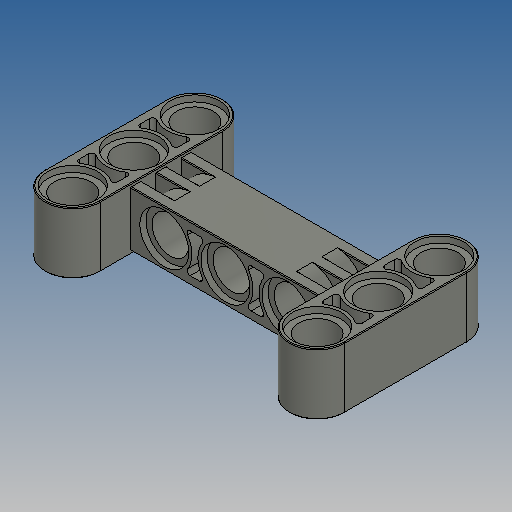
# Autodesk Inventor part: 14720-DkBluishGray
Saved by Autodesk Inventor 2025 (Build 290162010, 162A)
## iProperties
Created: 2012-03-21
Part Number: 14720-DkBluishGray
Document SubType Name: Modeling
Designer: D. Kohfeld
Density: 1.06 g/cm^3
Material: ABS Plastic
Mass: 2.24309 g
Surface Area: 36.022 cm^2
Volume: 2.11613 cm^3
Appearance: DkBluishGray
Author: D. Kohfeld
Autodesk Inventor part; units mm, degrees
ref_plane "YZ Plane" through (0, 0, 0) normal (1, 0, 0) x (0, 1, 0)
ref_plane "XZ Plane" through (0, 0, 0) normal (0, 1, 0) x (-1, 0, 0)
ref_plane "XY Plane" through (0, 0, 0) normal (0, 0, 1) x (1, 0, 0)
sketch "Sketch1" plane through (0, 0, 0) normal (0, 0, 1) x (1, 0, 0)
  line L0 (19.6, -8) -> (19.6, 8)
  line L1 (12.4, 8) -> (12.4, -8)
  arc A0 (19.6, 8) -> (12.4, 8) centre (16, 8) ccw
  arc A1 (12.4, -8) -> (19.6, -8) centre (16, -8) ccw
  circle A2 centre (16, 8) radius 3.2
  circle A3 centre (16, 8) radius 2.4
  line L2 (18.5456, 5.4544) -> (18.5456, 2.5456)
  line L3 (13.4544, 5.4544) -> (13.4544, 2.5456)
  arc A4 (13.4544, 5.4544) -> (18.5456, 5.4544) centre (16, 8) ccw
  arc A5 (18.5456, 2.5456) -> (13.4544, 2.5456) centre (16, 0) ccw
  circle A6 centre (16, 0) radius 3.2
  circle A7 centre (16, 0) radius 2.4
  line L4 (16, 8) -> (13.4544, 5.4544) construction
  circle A8 centre (16, -8) radius 3.2
  circle A9 centre (16, -8) radius 2.4
  line L5 (18.5456, -2.5456) -> (18.5456, -5.4544)
  line L6 (13.4544, -5.4544) -> (13.4544, -2.5456)
  arc A10 (13.4544, -2.5456) -> (18.5456, -2.5456) centre (16, 0) ccw
  arc A11 (18.5456, -5.4544) -> (13.4544, -5.4544) centre (16, -8) ccw
  point P0 (0, 0)
  point P1 (12.4, 0)
  dimension "d49" = 6.4
  dimension "d50" = 4.8
  dimension "d51" = 8
  dimension "d116" = 45
  dimension "d119" = 7.2
  dimension "d131" = 16
  constraints: 14 end point, 12 centre point, 12 point on circle, 9 coincident, 8 equal radius, 4 horizontal alignment, 4 tangent, 3 parallel, 3 vertical alignment, 2 vertical, 1 midpoint
  measures "d49" diameter of A2
  measures "d50" diameter of A3
  measures "d51" distance of A0.centre A5.centre
  measures "d116" angle of L4 L1
  measures "d119" diameter of A0
  measures "d131" distance of A6.centre point (0, 0)
extrude "Extrusion1" add sketch "Sketch1" along normal mid plane 8 contours A1 L1 A0 L0 | A2 | L2 A5 L3 A4 | A6 | A8 | L5 A11 L6 A10
sketch "Sketch6" plane through (0, 0, 4) normal (0, 0, 1) x (1, 0, 0)
  circle A0 centre (16, 8) radius 2.4 projected
  circle A1 centre (16, 8) radius 3.2 projected
  line L0 (18.5456, 5.4544) -> (18.5456, 2.5456) projected
  arc A2 (13.4544, 5.4544) -> (18.5456, 5.4544) centre (16, 8) ccw projected
  arc A3 (18.5456, 2.5456) -> (13.4544, 2.5456) centre (16, 0) ccw projected
  line L1 (13.4544, 5.4544) -> (13.4544, 2.5456) projected
  circle A4 centre (16, 0) radius 3.2 projected
  circle A5 centre (16, -8) radius 3.2 projected
  arc A6 (18.5456, -5.4544) -> (13.4544, -5.4544) centre (16, -8) ccw projected
  line L2 (13.4544, -5.4544) -> (13.4544, -2.5456) projected
  arc A7 (13.4544, -2.5456) -> (18.5456, -2.5456) centre (16, 0) ccw projected
  line L3 (18.5456, -2.5456) -> (18.5456, -5.4544) projected
extrude "Extrusion7" cut sketch "Sketch6" against normal blind 0.8 contours A0 | A1 | A4 | A5
extrude "Extrusion8" cut sketch "Sketch6" against normal blind 3.1 contours L0 A3 L1 A2 | A6 L2 A7 L3
mirror "Mirror5" about plane through (0, 0, 0) normal (0, 0, 1) of "Extrusion7", "Extrusion8"
fillet "Fillet2" radius 0.4 16 edges at (13.4544, 5.4544, 2.45) (13.4544, 2.5456, 2.45) (18.5456, 2.5456, 2.45) (18.5456, 5.4544, 2.45) (13.4544, -2.5456, 2.45) (18.5456, -5.4544, 2.45) (18.5456, -2.5456, 2.45) (13.4544, -5.4544, 2.45) (18.5456, -5.4544, -2.45) (18.5456, -2.5456, -2.45) (13.4544, -5.4544, -2.45) (13.4544, -2.5456, -2.45) (13.4544, 2.5456, -2.45) (13.4544, 5.4544, -2.45) (18.5456, 5.4544, -2.45) (18.5456, 2.5456, -2.45)
fillet "Fillet2" radius 0.1 8 edges at (12.4, 0, 4) (16, 11.6, 4) (19.6, 0, 4) (16, -11.6, 4) (16, 11.6, -4) (12.4, 0, -4) (16, -11.6, -4) (19.6, 0, -4)
sketch "Sketch11" plane through (0, 0, 0) normal (0, 1, 0) x (-1, 0, 0)
  line L0 (8, 3.6) -> (-8, 3.6)
  line L1 (-12.4, 1.111) -> (-12.4, -1.111)
  line L2 (-8, -3.6) -> (8, -3.6)
  line L3 (-12.4, -3.9) -> (-12.4, 3.9) projected
  line L4 (0, 3.6) -> (0, -3.6) construction
  arc A0 (-8, 3.6) -> (-8, -3.6) centre (-8, 0) ccw
  line L5 (-11.4243, 1.111) -> (-12.4, 1.111)
  line L6 (-11.4243, -1.111) -> (-12.4, -1.111)
  arc A1 (8, -3.6) -> (8, 3.6) centre (8, 0) ccw
  line L7 (11.4243, 1.111) -> (12.4, 1.111)
  line L8 (12.4, 1.111) -> (12.4, -1.111)
  line L9 (12.4, -1.111) -> (11.4243, -1.111)
  point P0 (-12.4, 0)
  point P1 (0, 0)
  point P2 (12.4, 0)
  point P3 (0, 0)
  dimension "d121" = 7.2
  dimension "d123" = 2.222
  dimension "d132" = 16
  constraints: 18 end point, 8 point on circle, 6 midpoint, 5 parallel, 4 perpendicular, 4 tangent, 3 horizontal alignment, 2 centre point, 2 point on line, 1 coincident
  measures "d121" distance between parallel lines of L2 L0
  measures "d123" distance between parallel lines of L6 L5
  measures "d132" distance of A1.centre A0.centre
extrude "Extrusion13" add sketch "Sketch11" along normal mid plane 8
sketch "Sketch12" plane through (0, -4, 0) normal (0, -1, 0) x (1, 0, 0)
  arc A0 (-8, 3.6) -> (-8, -3.6) centre (-8, 0) ccw projected
  arc A1 (8, -3.6) -> (11.4243, -1.111) centre (8, 0) ccw projected
  line L0 (11.4243, -1.111) -> (12.4, -1.111) projected
  circle A2 centre (8, 0) radius 2.4
  circle A3 centre (8, 0) radius 3.2
  circle A4 centre (0, 0) radius 2.4
  circle A5 centre (0, 0) radius 3.2
  circle A6 centre (-8, 0) radius 2.4
  circle A7 centre (-8, 0) radius 3.2
  line L1 (-8, 0) -> (0, 0) construction
  line L2 (0, 0) -> (8, 0) construction
  arc A8 (8, -3.6) -> (8, 3.6) centre (8, 0) ccw projected
  arc A9 (-8, 3.6) -> (-8, -3.6) centre (-8, 0) ccw projected
  line L3 (-8, -3.6) -> (8, -3.6) projected
  line L4 (-5.4544, 2.5456) -> (-2.5456, 2.5456)
  line L5 (-5.4544, -2.5456) -> (-2.5456, -2.5456)
  line L6 (2.5456, 2.5456) -> (5.4544, 2.5456)
  line L7 (2.5456, -2.5456) -> (5.4544, -2.5456)
  arc A10 (-5.4544, -2.5456) -> (-5.4544, 2.5456) centre (-8, 0) ccw
  arc A11 (-2.5456, 2.5456) -> (-2.5456, -2.5456) centre (0, 0) ccw
  arc A12 (2.5456, -2.5456) -> (2.5456, 2.5456) centre (0, 0) ccw
  arc A13 (5.4544, 2.5456) -> (5.4544, -2.5456) centre (8, 0) ccw
  line L8 (-8, 0) -> (-5.4544, 2.5456) construction
  point P0 (-11.4243, -1.111)
  point P1 (11.4243, 1.111)
  point P2 (-11.4243, 1.111)
  point P3 (-6.8156, -3.3996)
  dimension "d124" = 4.8
  dimension "d125" = 6.4
  dimension "d126" = 45
  constraints: 14 end point, 10 centre point, 9 coincident, 8 equal radius, 8 point on circle, 5 parallel, 3 equal length, 1 collinear, 1 horizontal alignment, 1 other
  measures "d124" diameter of A2
  measures "d125" diameter of A3
  measures "d126" angle of L1 L8
extrude "Extrusion14" cut sketch "Sketch12" against normal through all contours A2 | A4 | A6
extrude "Extrusion15" cut sketch "Sketch12" against normal blind 3.2 contours L4 A11 L5 A10 | L6 A13 L7 A12
extrude "Extrusion16" cut sketch "Sketch12" against normal blind 0.8 contours A3 | A5 | A7
sketch "Sketch16" plane through (-8, 4, 3.6) normal (0, 0, 1) x (1, 0, 0)
  line L0 (16, -8) -> (16, 0) projected
  line L1 (20.4, 4) -> (20.4, -12) construction
  line L2 (16, 0) -> (20.4, 0)
  line L3 (20.4, 0) -> (20.4, -1.4)
  line L4 (20.4, -1.4) -> (16, -1.4)
  line L5 (16, -1.4) -> (16, 0)
  line L6 (16, -3.3) -> (20.4, -3.3)
  line L7 (20.4, -3.3) -> (20.4, -4.7)
  line L8 (20.4, -4.7) -> (16, -4.7)
  line L9 (16, -4.7) -> (16, -3.3)
  line L10 (16, -8) -> (20.4, -8)
  line L11 (20.4, -8) -> (20.4, -6.6)
  line L12 (20.4, -6.6) -> (16, -6.6)
  line L13 (16, -6.6) -> (16, -8)
  line L14 (0, 0) -> (0, -8) projected
  line L15 (-4.4, -8) -> (-4.4, 0) construction
  line L16 (0, 0) -> (-4.4, 0)
  line L17 (-4.4, 0) -> (-4.4, -1.4)
  line L18 (-4.4, -1.4) -> (0, -1.4)
  line L19 (0, -1.4) -> (0, 0)
  line L20 (0, -3.3) -> (-4.4, -3.3)
  line L21 (-4.4, -3.3) -> (-4.4, -4.7)
  line L22 (-4.4, -4.7) -> (0, -4.7)
  line L23 (0, -4.7) -> (0, -3.3)
  line L24 (0, -8) -> (-4.4, -8)
  line L25 (-4.4, -8) -> (-4.4, -6.6)
  line L26 (-4.4, -6.6) -> (0, -6.6)
  line L27 (0, -6.6) -> (0, -8)
  point P0 (8, -4)
  point P1 (16, -4)
  point P2 (0, -4)
  dimension "d127" = 1.4
  constraints: 48 end point, 12 parallel, 8 point on line, 6 horizontal, 6 perpendicular, 5 equal length, 4 midpoint
  measures "d127" distance between parallel lines of L8 L6
extrude "Extrusion20" add sketch "Sketch16" against normal up to next
fillet "Fillet4" radius 0.4 8 edges at (-5.4544, -2.4, 2.5456) (-2.5456, -2.4, 2.5456) (-5.4544, -2.4, -2.5456) (-2.5456, -2.4, -2.5456) (2.5456, -2.4, 2.5456) (5.4544, -2.4, 2.5456) (2.5456, -2.4, -2.5456) (5.4544, -2.4, -2.5456)
mirror "Mirror6" about plane through (0, 0, 0) normal (0, 1, 0) of "Extrusion15", "Extrusion16", "Fillet4"
mirror "Mirror4" about plane through (0, 0, 0) normal (0, 0, 1) of "Extrusion20"
mirror "Mirror3" about plane through (0, 0, 0) normal (1, 0, 0) of "Extrusion7", "Extrusion1", "Extrusion8", "Fillet2", "Mirror5"
fillet "Fillet5" radius 0.1 20 edges at (0, -4, 3.6) (0, 4, 3.6) (-10.2, 2.6, 3.6) (-10.2, 0.7, 3.6) (-10.2, -0.7, 3.6) (-10.2, -2.6, 3.6) (10.2, 2.6, 3.6) (10.2, 0.7, 3.6) (10.2, -0.7, 3.6) (10.2, -2.6, 3.6) (0, 4, -3.6) (10.2, 2.6, -3.6) (10.2, 0.7, -3.6) (10.2, -0.7, -3.6) (10.2, -2.6, -3.6) (0, -4, -3.6) (-10.2, 2.6, -3.6) (-10.2, 0.7, -3.6) (-10.2, -0.7, -3.6) (-10.2, -2.6, -3.6)
equation "\"lf\" = 0.1"
equation "\"tf\" = 0.4"
body "Solid1"
